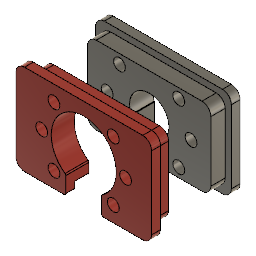
BallScrewKeyholeFacePlate (Autodesk Fusion 360 design; units mm, degrees)
Autodesk Fusion 360 part; units mm, degrees
note: some values were not read from the file. Set by a fixed rule: which face or edge a step refers to.
sketch "Sketch1" plane through (0, 0, 0) normal (0, 1, 0) x (1, 0, 0)
  line L0 (-38.1, -25.4) -> (38.1, -25.4)
  line L1 (38.1, -25.4) -> (38.1, 25.4)
  line L2 (38.1, 25.4) -> (-38.1, 25.4)
  line L3 (-38.1, 25.4) -> (-38.1, -25.4)
  line L4 (0, -25.4) -> (0, 25.4) construction
  line L5 (35.1, 22.4) -> (-35.1, 22.4)
  line L6 (-35.1, 22.4) -> (-35.1, -22.4)
  line L7 (-35.1, -22.4) -> (35.1, -22.4)
  line L8 (35.1, -22.4) -> (35.1, 22.4)
  circle A0 centre (0, 0) radius 18
  circle A1 centre (0, 0) radius 23.502 construction
  circle A2 centre (23.502, 0) radius 3.3058
  line L9 (0, 0) -> (23.502, 0) construction
  line L10 (0, 25.4) -> (-10, 25.4)
  line L11 (-10, 25.4) -> (-10, 25.3999)
  line L12 (10, 25.4) -> (10, 25.3999)
  circle A3 centre (0, 0) radius 11
  line L13 (-10, 25.3999) -> (-10, 4.5826)
  circle A4 centre (16.6185, 16.6185) radius 3.3058
  circle A5 centre (-16.6185, 16.6185) radius 3.3058
  circle A6 centre (-23.502, 0) radius 3.3058
  circle A7 centre (-16.6185, -16.6185) radius 3.3058
  circle A8 centre (16.6185, -16.6185) radius 3.3058
  line L14 (10, 25.3999) -> (10, 4.5826)
  dimension "d15" = 76.2
  dimension "d16" = 50.8
  dimension "d18" = 36
  dimension "d19" = 47.0041
  dimension "d20" = 6.6116
  dimension "d31" = 10
  dimension "d41" = 22
  dimension "d47" = 360
  constraint horizontal L0
  constraint vertical L1
  constraint horizontal L2
  constraint vertical L3
  constraint coincident L0 L4.start
  constraint midpoint L2 L4.end
  constraint vertical L4
  constraint midpoint A0.centre L4
  constraint coincident A0.centre A1.centre
  constraint coincident A1 A2.centre
  constraint coincident A2.centre L9.end
  constraint horizontal L9
  constraint horizontal L10
  constraint vertical L11
  constraint symmetric L4 L10.end L12.start
  constraint symmetric L4 L11.end L12.end
  constraint concentric A1 A3
  constraint coincident A3 L13.end
  constraint parallel L11 L13
  constraint symmetric L4 L13.end L14.end
  measures "d15" distance of L0.start L0.end
  measures "d16" distance of L0.start L2.end
  measures "d18" diameter of A0
  measures "d19" diameter of A1
  measures "d20" diameter of A2
  measures "d31" distance of L4.end L10.end
  measures "d41" diameter of A3
extrude "Extrude1" add sketch "Sketch1" along normal blind 5 contours L0 L1 L2 L3 L5 L6 L7 L8 L13 L14 | L5 L6 L7 L8 A0 L13 L14 makes body 1
extrude "Extrude2" add sketch "Sketch1" along normal blind 13 contours L5 L6 L7 L8 A0 L13 L14 bodies 1
move_face "OffsetFaces1" offset -0.5 5 faces at (-11.7, 7.6667, 22.4) (-35.1, 7.6667, -7.4667) (26.7333, 10.3333, -22.4) (-18.3667, 10.3333, -22.4) (35.1, 7.6667, 7.4667) on bodies 1
fillet "Fillet2" radius 5 8 edges at (-34.6, 9, 21.9) (-38.1, 2.5, 25.4) (-38.1, 2.5, -25.4) (-34.6, 9, -21.9) (34.6, 9, -21.9) (38.1, 2.5, -25.4) (34.6, 9, 21.9) (38.1, 2.5, 25.4) on bodies 1
move_face "OffsetFaces2" offset -0.15 1 faces at (-11.4058, 8.6667, -13.9251) on bodies 1
extrude "Extrude4" add sketch "Sketch1" along normal blind 5 separate body contours L0 L1 L2 L3 L5 L6 L7 L8 L13 L14 | L5 L6 L7 L8 A0 L13 L14 | A0 A3 L13 L14 picked at (-14.0229, 6.9084) makes body 2
extrude "Extrude5" add sketch "Sketch1" along normal blind 13 contours L5 L6 L7 L8 A0 L13 L14 | A0 A3 L13 L14 picked at (-14.0229, 6.9084) bodies 2
move_face "OffsetFaces3" offset -0.5 5 faces at (-11.7, 7.6667, 22.4) (-35.1, 7.6667, -7.4667) (35.1, 7.6667, 7.4667) (26.7333, 10.3333, -22.4) (-18.3667, 10.3333, -22.4) on bodies 2
move_body "Move1" bodies 2 to x (-1, 0, 0) y (0, -1, 0) z (0, 0, 1) at (0.5097, 49.7115, -0.0036)
move_body "Align1" bodies 1 to x (1, 0, 0) y (0, 1, 0) z (0, 0, 1) at (0.5097, 0, 0)
fillet "Fillet3" radius 5 8 edges at (-37.5903, 47.2115, 25.3964) (-34.0903, 40.7115, 21.8964) (-34.0903, 40.7115, -21.9036) (-37.5903, 47.2115, -25.4036) (38.6097, 47.2115, 25.3964) (35.1097, 40.7115, 21.8964) (35.1097, 40.7115, -21.9036) (38.6097, 47.2115, -25.4036) on bodies 2
fillet "Fillet4" radius 1 10 edges at (-9.4903, 6.5, -15.1467) (-9.4903, 2.5, -25.4) (-9.4903, 9, -21.9) (10.5097, 2.5, -25.4) (10.5097, 47.2115, -25.4036) (10.5097, 40.7115, -21.9036) (-9.4903, 47.2115, -25.4036) (-9.4903, 40.7115, -21.9036) (-9.4903, 43.2115, -4.5862) (10.5097, 43.2115, -4.5862) on bodies 1 2
copy_body "Body->Comp2" bodies 1 removing the originals makes body 3 in component "Ballscrew Plate"
copy_body "Body->Comp3" bodies 2 removing the originals makes body 4 in component "Filler Plate"
component "Ballscrew Plate" placed x (1, 0, 0) y (0, 1, 0) z (0, 0, 1) at (0, 0, 0)
component "Filler Plate" placed x (1, 0, 0) y (0, 1, 0) z (0, 0, 1) at (0, 0, 0)
equation "steelWide_Ref = 76.2 mm"
equation "steelNarrow_Ref = 50.8 mm"
equation "steelThick_Ref = 3 mm"
equation "steelRadius_Ref = 5 mm"
equation "d15 = steelWide_Ref"
equation "d16 = steelNarrow_Ref"
equation "d17 = -steelThick_Ref"
equation "d18 = ( BallScrewDiameter * 2 ) - 4 mm"
equation "d19 = ( BallScrewDiameter + 0.9 mm ) * 2.249"
equation "d20 = ( BallScrewDiameter + 4 mm ) / 3.63"
equation "d23 = nutPlate"
equation "d29 = steelRadius_Ref"
equation "d31 = BallScrewDiameter / 2"
equation "nutPlate = 13 mm"
equation "d41 = BallScrewDiameter + 2 mm"
equation "d49 = steelRadius_Ref"
equation "BallScrewDiameter = 20 mm"
